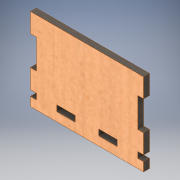
# Autodesk Inventor part: HolderDCDC
Saved by Autodesk Inventor 2019 (Build 230136000, 136)
## iProperties
Created: 2021-01-03
Part Number: HolderDCDC
Material: Типовые
Document SubType Name: Modeling
Designer: Professional
Density: 1 g/cm^3
Appearance: Вишневое дерево — натуральный — со слабым глянцем
Author: Professional
Autodesk Inventor part; units mm, degrees
ref_plane "YZ Plane" through (0, 0, 0) normal (1, 0, 0) x (0, 1, 0)
ref_plane "XZ Plane" through (0, 0, 0) normal (0, 1, 0) x (-1, 0, 0)
ref_plane "XY Plane" through (0, 0, 0) normal (0, 0, 1) x (1, 0, 0)
sketch "Эскиз1" plane through (0, 0, 0) normal (0, 0, 1) x (1, 0, 0)
  line L0 (0, 0) -> (-38.5, 0)
  line L1 (-38.5, 0) -> (-38.5, 6)
  line L2 (-38.5, 6) -> (-34.5, 6)
  line L3 (-34.5, 6) -> (-34.5, 10)
  line L4 (-34.5, 10) -> (-38.5, 10)
  line L5 (-38.5, 10) -> (-38.5, 23)
  line L6 (-38.5, 23) -> (-34.5, 23)
  line L7 (-34.5, 23) -> (-34.5, 43)
  line L8 (-34.5, 43) -> (-38.5, 43)
  line L9 (-38.5, 43) -> (-38.5, 56)
  line L10 (-38.5, 56) -> (0, 56)
  line L11 (0, 56) -> (0, 0)
  line L12 (0, 0) -> (38.5, 0)
  line L13 (38.5, 0) -> (38.5, 6)
  line L14 (38.5, 6) -> (34.5, 6)
  line L15 (34.5, 6) -> (34.5, 10)
  line L16 (34.5, 10) -> (38.5, 10)
  line L17 (38.5, 10) -> (38.5, 23)
  line L18 (38.5, 23) -> (34.5, 23)
  line L19 (34.5, 23) -> (34.5, 43)
  line L20 (34.5, 43) -> (38.5, 43)
  line L21 (38.5, 43) -> (38.5, 56)
  line L22 (38.5, 56) -> (0, 56)
  line L23 (-20.5, 10) -> (-8, 10)
  line L24 (-8, 10) -> (-8, 6)
  line L25 (-8, 6) -> (-20.5, 6)
  line L26 (-20.5, 6) -> (-20.5, 10)
  line L27 (20.5, 10) -> (8, 10)
  line L28 (8, 10) -> (8, 6)
  line L29 (8, 6) -> (20.5, 6)
  line L30 (20.5, 6) -> (20.5, 10)
  dimension "d0" = 4
  dimension "d1" = 6
  dimension "d2" = 4
  dimension "d3" = 46
  dimension "d4" = 20
  dimension "d5" = 13
  dimension "d6" = 13
  dimension "d7" = 77
  dimension "d10" = 12.5
  dimension "d11" = 16
  constraints: 62 end point, 14 symmetric about line, 9 perpendicular, 8 point on line, 3 horizontal, 2 horizontal alignment, 2 parallel, 2 vertical alignment
  measures "d0" distance between parallel lines of L1 L3
  measures "d1" distance between parallel lines of L0 L2
  measures "d2" distance between parallel lines of L4 L2
  measures "d3" distance between parallel lines of L10 L4
  measures "d4" distance between parallel lines of L6 L8
  measures "d5" distance between parallel lines of L10 L8
  measures "d6" distance between parallel lines of L4 L6
  measures "d7" distance between parallel lines of L21 L9
  measures "d10" distance between parallel lines of L24 L26
  measures "d11" distance between parallel lines of L28 L24
extrude "Выдавливание1" add sketch "Эскиз1" along normal blind 4
